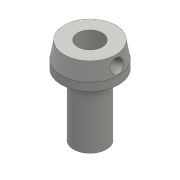
# Autodesk Inventor part: Midle
Saved by Autodesk Inventor 2016 (Build 200138000, 138)
## iProperties
Created: 2020-10-21
Part Number: Midle
Material: Generic
Document SubType Name: Modeling
Designer: extract
Density: 1 g/cm^3
Appearance: Default
Author: extract
Autodesk Inventor part; units mm, degrees
ref_plane "YZ Plane" through (0, 0, 0) normal (1, 0, 0) x (0, 1, 0)
ref_plane "XY Plane" through (0, 0, 0) normal (0, 0, 1) x (1, 0, 0)
sketch "Sketch1" plane through (0, 0, 0) normal (0, 0, 1) x (1, 0, 0)
  circle A0 centre (0, 0) radius 10
  dimension "d0" = 20
  constraints: 1 centre point, 1 coincident
  measures "d0" diameter of A0
extrude "Extrusion1" add sketch "Sketch1" along normal blind 38
sketch "Sketch2" plane through (0, 0, 38) normal (0, 0, 1) x (1, 0, 0)
  circle A0 centre (0, 0) radius 17.5
  dimension "d3" = 35
  constraints: 1 centre point, 1 coincident
  measures "d3" diameter of A0
extrude "Extrusion2" add sketch "Sketch2" along normal blind 5
sketch "Sketch3" plane through (0, 0, 43) normal (0, 0, 1) x (1, 0, 0)
  circle A0 centre (0, 0) radius 17.5 projected
extrude "Extrusion3" add sketch "Sketch3" along normal blind 10 draft -10
sketch "Sketch4" plane through (0, 0, 53) normal (0, 0, 1) x (1, 0, 0)
  circle A0 centre (0, 0) radius 7.5
  dimension "d9" = 15
  constraints: 1 centre point, 1 coincident
  measures "d9" diameter of A0
extrude "Extrusion4" cut sketch "Sketch4" against normal through all
ref_plane "Work Plane1" through (15.7367, 0, 53) normal (0.9848, 0, 0.1736) x (0, 1, 0)
sketch "Sketch6" plane through (15.7367, 0, 53) normal (0.9848, 0, 0.1736) x (0, 1, 0)
  circle A0 centre (0, -5.4313) radius 4
  point P0 (0, -49.4622)
  dimension "d12" = 8
  constraints: 1 centre point
  measures "d12" diameter of A0
extrude "Extrusion5" cut sketch "Sketch6" against normal blind 13.25
body "Solid1"
